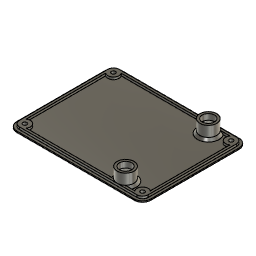
MainCaseTop (Autodesk Fusion 360 design; units mm, degrees)
Autodesk Fusion 360 part; units mm, degrees
sketch "Skizze1" plane through (0, 0, 0) normal (0, 0, 1) x (1, 0, 0)
  line L0 (0, 0) -> (115, 0)
  line L1 (115, 0) -> (115, 90)
  line L2 (115, 90) -> (0, 90)
  line L3 (0, 90) -> (0, 0)
  dimension "d1" = 115
  dimension "d2" = 90
  constraint horizontal L0
  constraint vertical L1
  constraint horizontal L2
  constraint vertical L3
  constraint coincident L0.start L3.end
  measures "d1" distance of L0.start L0.end
  measures "d2" distance of L0.end L1.end
extrude "Extrusion1" add sketch "Skizze1" along normal blind 1
fillet "Abrundung1" radius 7 4 edges at (0, 0, 0.5) (0, 90, 0.5) (115, 0, 0.5) (115, 90, 0.5)
sketch "Skizze4" plane through (0, 0, 1) normal (0, 0, 1) x (-1, 0, 0)
  arc A0 (-115, -83) -> (-108, -90) centre (-108, -83) ccw
  line L0 (-108, -90) -> (-7, -90)
  arc A1 (-7, -90) -> (0, -83) centre (-7, -83) ccw
  line L1 (0, -83) -> (0, -7)
  arc A2 (0, -7) -> (-7, 0) centre (-7, -7) ccw
  line L2 (-7, 0) -> (-108, 0)
  arc A3 (-108, 0) -> (-115, -7) centre (-108, -7) ccw
  line L3 (-115, -7) -> (-115, -83)
  arc A4 (-7, -90) -> (0, -83) centre (-7, -83) ccw
  arc A5 (-115, -83) -> (-108, -90) centre (-108, -83) ccw
  arc A6 (-108, 0) -> (-115, -7) centre (-108, -7) ccw
  arc A7 (0, -7) -> (-7, 0) centre (-7, -7) ccw
  circle A8 centre (-7, -83) radius 4.8
  circle A9 centre (-108, -83) radius 4.8
  circle A10 centre (-108, -7) radius 4.8
  circle A11 centre (-7, -7) radius 4.8
  dimension "d19" = 9.6
  dimension "d20" = 9.6
  dimension "d21" = 9.6
  dimension "d22" = 9.6
  constraint concentric A4 A8
  constraint concentric A5 A9
  constraint concentric A6 A10
  constraint concentric A7 A11
  measures "d19" diameter of A11
  measures "d20" diameter of A10
  measures "d21" diameter of A9
  measures "d22" diameter of A8
extrude "Extrusion3" add sketch "Skizze4" along normal blind 2 contours A8 | A9 | A10 | A11
sketch "Skizze9" plane through (0, 0, 3) normal (0, 0, 1) x (-1, 0, 0)
  circle A0 centre (-7, -7) radius 4.8
  circle A1 centre (-7, -83) radius 4.8
  circle A2 centre (-108, -83) radius 4.8
  circle A3 centre (-108, -7) radius 4.8
  point P0 (-7, -83)
  point P1 (-108, -83)
  point P2 (-108, -7)
  point P3 (-7, -7)
  constraint coincident P0 A1.centre
  constraint coincident P1 A2.centre
  constraint coincident P2 A3.centre
  constraint coincident P3 A0.centre
hole "Bohrung4" at (7, 83, 3) at (7, 7, 3) at (108, 83, 3) at (108, 7, 3) direction (0, 0, -1) diameter 3.5 depth 12 tip angle 180
sketch "Skizze6" plane through (0, 0, 1) normal (0, 0, 1) x (-1, 0, 0)
  circle A0 centre (-7, -7) radius 4.8
  circle A1 centre (-7, -83) radius 4.8
  circle A2 centre (-108, -7) radius 4.8
  circle A3 centre (-108, -83) radius 4.8
  arc A4 (-115, -83) -> (-108, -90) centre (-108, -83) ccw
  line L0 (-108, -90) -> (-7, -90)
  arc A5 (-7, -90) -> (0, -83) centre (-7, -83) ccw
  line L1 (0, -83) -> (0, -7)
  arc A6 (0, -7) -> (-7, 0) centre (-7, -7) ccw
  line L2 (-7, 0) -> (-108, 0)
  arc A7 (-108, 0) -> (-115, -7) centre (-108, -7) ccw
  line L3 (-115, -7) -> (-115, -83)
  circle A8 centre (-7, -83) radius 4.8
  circle A9 centre (-108, -83) radius 4.8
  circle A10 centre (-108, -7) radius 4.8
  circle A11 centre (-7, -7) radius 4.8
  line L4 (-2.2, -7) -> (-2.2, -82.9976)
  line L5 (-7, -87.8) -> (-108, -87.8)
  line L6 (-111.8987, -85.8) -> (-10.8987, -85.8)
  line L7 (-112.8, -83) -> (-112.8, -7)
  line L8 (-110.8, -10.8987) -> (-110.8, -79.1013)
  line L9 (-108, -2.2) -> (-7, -2.2)
  line L10 (-10.8987, -4.2) -> (-111.8987, -4.2)
  line L11 (-4.2, -79.1013) -> (-4.2, -10.8987)
  circle A12 centre (-7, -83) radius 1.75
  circle A13 centre (-108, -83) radius 1.75
  circle A14 centre (-108, -7) radius 1.75
  circle A15 centre (-7, -7) radius 1.75
  dimension "d42" = 2
  dimension "d43" = 2
  dimension "d44" = 2
  dimension "d45" = 2
  constraint coincident A11 L4.start
  constraint coincident A8 L4.end
  constraint tangent A1 L4
  constraint tangent A0 L4
  constraint coincident A8 L5.start
  constraint coincident A9 L5.end
  constraint parallel L0 L5
  constraint coincident A3 L6.start
  constraint coincident A8 L6.end
  constraint parallel L5 L6
  constraint coincident A9 L7.start
  constraint coincident A10 L7.end
  constraint perpendicular L6 L7
  constraint coincident A10 L8.start
  constraint coincident A9 L8.end
  constraint parallel L7 L8
  constraint coincident A10 L9.start
  constraint coincident A11 L9.end
  constraint perpendicular L8 L9
  constraint coincident A11 L10.start
  constraint coincident A10 L10.end
  constraint parallel L9 L10
  constraint tangent A2 L9
  constraint tangent A10 L7
  constraint tangent A9 L5
  constraint coincident A8 L11.start
  constraint coincident A11 L11.end
  constraint parallel L4 L11
  measures "d42" distance of L5 L6
  measures "d43" distance of L7 L8
  measures "d44" distance of L9 L10
  measures "d45" distance of L4 L11
extrude "Extrusion4" add sketch "Skizze6" along normal blind 2 contours A0 A1 A8 A11 L4 L11 | A0 A2 A10 A11 L9 L10 | A1 A3 A8 A9 L5 L6 | A2 A3 A9 A10 L7 L8
sketch "Skizze7" plane through (0, 0, 1) normal (0, 0, 1) x (-1, 0, 0)
  arc A0 (-4.2, -79.1013) -> (-10.8987, -85.8) centre (-7, -83) ccw
  arc A1 (-10.8987, -4.2) -> (-4.2, -10.8987) centre (-7, -7) ccw
  circle A2 centre (-90.9, -80.5) radius 7.25
  circle A3 centre (-90.9, -9.5) radius 7.25
  line L0 (-7, 0) -> (-108, 0)
  line L1 (-108, -90) -> (-7, -90)
  line L2 (-104.1013, -85.8) -> (-10.8987, -85.8)
  arc A4 (-104.1013, -85.8) -> (-110.8, -79.1013) centre (-108, -83) ccw
  arc A5 (-110.8, -10.8987) -> (-104.1013, -4.2) centre (-108, -7) ccw
  line L3 (-4.2, -79.1013) -> (-4.2, -10.8987)
  line L4 (-10.8987, -4.2) -> (-104.1013, -4.2)
  line L5 (-110.8, -10.8987) -> (-110.8, -79.1013)
  dimension "d34" = 14.5
  dimension "d35" = 14.5
  dimension "d36" = 90.9
  dimension "d37" = 71
  dimension "d38" = 9.5
  dimension "d39" = 9.5
  constraint vertical A2.centre A3.centre
  measures "d34" diameter of A3
  measures "d35" diameter of A2
  measures "d36" horizontal distance of origin A3.centre
  measures "d37" distance of A2.centre A3.centre
  measures "d38" distance of A3.centre L0
  measures "d39" distance of A2.centre L1
extrude "Extrusion5" add sketch "Skizze7" along normal blind 11 contours A2 L2 | A2 L2 | A3 L4 | A3 L4
sketch "Skizze8" plane through (0, 0, 12) normal (0, 0, 1) x (-1, 0, 0)
  circle A0 centre (-90.9, -80.5) radius 7.25
  circle A1 centre (-90.9, -9.5) radius 7.25
  point P0 (-90.9, -80.5)
  point P1 (-90.9, -9.5)
  constraint coincident P0 A0.centre
  constraint coincident P1 A1.centre
hole "Bohrung3" at (90.9, 80.5, 12) at (90.9, 9.5, 12) direction (0, 0, -1) diameter 10.5 depth 12 tip angle 180
chamfer "Fase1" distance 2 distance2 7 1 edges at (86.0053, 7.6015, 0) measured on face at (34.4568, 55.7422, 0)
chamfer "Fase1" distance 2 distance2 7 1 edges at (86.0053, 78.6015, 0) measured on face at (34.4568, 55.7422, 0)
chamfer "Fase2" distance 2 angle 45 2 edges at (90.9, 73.25, 1) (90.9, 16.75, 1)
equation "d38 = d39"
